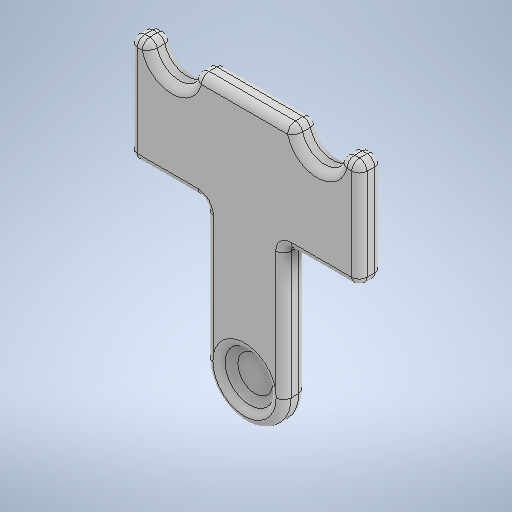
# Autodesk Inventor part: Screw_Aligner_FTC_LapCnrBkt
Saved by Autodesk Inventor 2025.1 (Build 291241000, 241)
## iProperties
Created: 2024-08-19
Part Number: Screw_Aligner_FTC_LapCnrBkt
Material: Generic
Document SubType Name: Modeling
Designer: shubh
Density: 1 g/cm^3
Appearance: Default
Author: shubh
Autodesk Inventor part; units mm, degrees
ref_plane "YZ Plane" through (0, 0, 0) normal (1, 0, 0) x (0, 1, 0)
ref_plane "XZ Plane" through (0, 0, 0) normal (0, 1, 0) x (-1, 0, 0)
ref_plane "XY Plane" through (0, 0, 0) normal (0, 0, 1) x (1, 0, 0)
sketch "Sketch1" plane through (0, 0, 0) normal (0, 0, 1) x (1, 0, 0)
  line L0 (0, 0) -> (15, 0)
  line L1 (15, 0) -> (15, 7)
  line L2 (0, 7) -> (0, 0)
  line L3 (7.5, 0) -> (7.5, -14.9285) construction
  circle A0 centre (7.5, -8.7962) radius 2.54 construction
  line L4 (4.96, 0) -> (4.96, -8.7962)
  line L5 (10.04, 0) -> (10.04, -8.7962)
  arc A1 (4.96, -8.7962) -> (10.04, -8.7962) centre (7.5, -8.7962) ccw
  line L6 (7.5, 7) -> (7.5, 0) construction
  line L7 (0, 3.5) -> (15, 3.5) construction
  arc A2 (1.25, 7) -> (4.25, 7) centre (2.75, 7) ccw
  arc A3 (10.75, 7) -> (13.75, 7) centre (12.25, 7) ccw
  line L8 (0, 7) -> (1.25, 7)
  line L9 (4.25, 7) -> (10.75, 7)
  line L10 (13.75, 7) -> (15, 7)
  dimension "d0" = 15
  dimension "d1" = 7
  dimension "d2" = 5.08
  dimension "d3" = 3
  dimension "d4" = 1.5
  dimension "d5" = 12.5
  dimension "d6" = 0
  dimension "d7" = 15.7962
  constraints: 22 end point, 8 point on circle, 4 centre point, 3 midpoint, 3 perpendicular, 3 point on line, 3 symmetric about line, 3 tangent, 2 collinear, 2 horizontal, 1 parallel, 1 vertical, 1 other
  measures "d0" distance of L2.start L1.end
  measures "d1" distance of L1.end L0.end
  measures "d2" diameter of A0
  measures "d3" distance of L8.end L9.start
  measures "d4" radius of A2
  measures "d5" distance of L10.start L8.end
  measures "d6" distance from line of L10.start L9
  measures "d7" distance from line of L5.end L9
extrude "Extrusion1" add sketch "Sketch1" along normal blind 1.5
sketch "Sketch2" plane through (0, 0, 1.5) normal (0, 0, 1) x (1, 0, 0)
  line L0 (15, 7) -> (13.75, 7) construction
  arc A0 (10.75, 7) -> (13.75, 7) centre (12.25, 7) ccw construction
  line L1 (10.75, 7) -> (4.25, 7) construction
  arc A1 (1.25, 7) -> (4.25, 7) centre (2.75, 7) ccw construction
  line L2 (1.25, 7) -> (0, 7) construction
  line L3 (0, 7) -> (0, 0) construction
  line L4 (0, 0) -> (4.96, 0) construction
  line L5 (4.96, 0) -> (4.96, -8.7962) construction
  arc A2 (4.96, -8.7962) -> (10.04, -8.7962) centre (7.5, -8.7962) ccw construction
  line L6 (10.04, -8.7962) -> (10.04, 0) construction
  line L7 (10.04, 0) -> (15, 0) construction
  line L8 (15, 0) -> (15, 7) construction
  line L9 (7.5, -8.7962) -> (7.5, 0) construction
  line L10 (7.5, -8.7962) -> (7.5, -11.3362) construction
  circle A3 centre (7.5, -8.7962) radius 1.5875
  dimension "d10" = 3.175
  constraints: 4 end point, 1 centre point, 1 coincident, 1 point on circle, 1 vertical
  measures "d10" diameter of A3
extrude "Extrusion2" cut sketch "Sketch2" against normal blind 0.7
fillet "Fillet1" radius 0.5 36 edges at (4.96, 0, 0.75) (2.48, 0, 1.5) (2.48, 0, 0) (0, 0, 0.75) (0, 3.5, 1.5) (0, 3.5, 0) (2.75, 5.5, 1.5) (2.75, 5.5, 0) (1.25, 7, 0.75) (0.625, 7, 1.5) (0.625, 7, 0) (0, 7, 0.75) (12.25, 5.5, 1.5) (14.375, 7, 1.5) (12.25, 5.5, 0) (13.75, 7, 0.75) (14.375, 7, 0) (7.5, 7, 1.5) (4.25, 7, 0.75) (10.75, 7, 0.75) (7.5, 7, 0) (15, 3.5, 1.5) (12.52, 0, 1.5) (7.5, -11.3362, 0) (10.04, -4.3981, 0) (4.96, -4.3981, 0) (7.5, -11.3362, 1.5) (10.04, -4.3981, 1.5) (4.96, -4.3981, 1.5) (5.9125, -8.7962, 1.5) (5.9125, -8.7962, 0.8) (10.04, 0, 0.75) (12.52, 0, 0) (15, 0, 0.75) (15, 7, 0.75) (15, 3.5, 0)
body "Solid1"
